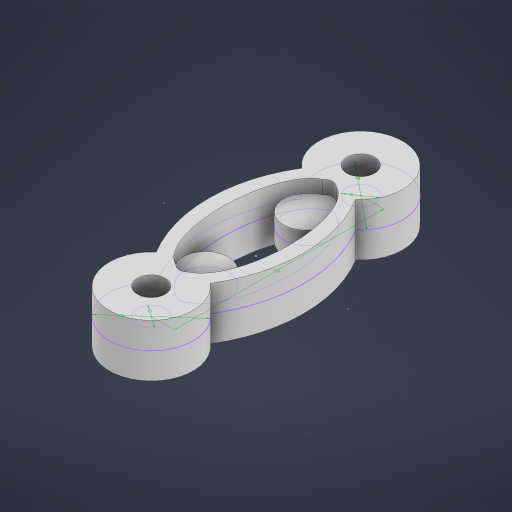
# Autodesk Inventor part: Part_A
Saved by Autodesk Inventor 2024.3 (Build 283343000, 343)
## iProperties
Created: 2025-07-11
Part Number: Part_A
Material: Generic
Document SubType Name: Modeling
Designer: LeoFB
Density: 1 g/cm^3
Appearance: Default
Author: LeoFB
Autodesk Inventor part; units mm, degrees
ref_plane "YZ Plane" through (0, 0, 0) normal (1, 0, 0) x (0, 1, 0)
ref_plane "XZ Plane" through (0, 0, 0) normal (0, 1, 0) x (-1, 0, 0)
ref_plane "XY Plane" through (0, 0, 0) normal (0, 0, 1) x (1, 0, 0)
sketch "Sketch1" plane through (0, 0, 0) normal (0, 1, 0) x (-1, 0, 0)
  circle A0 centre (0, 60) radius 8
  circle A1 centre (0, -60) radius 8
  arc A2 (15.4616, 41.6441) -> (-15.4616, 41.6441) centre (0, 60) ccw
  arc A3 (-15.4616, -41.6441) -> (15.4616, -41.6441) centre (0, -60) ccw
  arc A4 (15.4616, -41.6441) -> (15.4616, 41.6441) centre (-52.6044, 0) ccw
  arc A5 (-15.4616, 41.6441) -> (-15.4616, -41.6441) centre (52.6044, 0) ccw
  arc A6 (3.8493, 42.1449) -> (-3.8493, 42.1449) centre (0, 38.9538) ccw
  arc A7 (-3.8493, -42.1449) -> (3.8493, -42.1449) centre (0, -38.9538) ccw
  ellipse E0 centre (0, 0) end of major axis (0, 43.0192) minor radius 19.1905 (3.8493, -42.1449) -> (3.8493, 42.1449) ccw
  ellipse E1 centre (0, 0) end of major axis (0, 43.0192) minor radius 19.1905 (-3.8493, 42.1449) -> (-3.8493, -42.1449) ccw
  arc A8 (12.3481, -32.9308) -> (-12.3481, -32.9308) centre (0, -28.8656) ccw
  arc A9 (-12.3481, 32.9308) -> (12.3481, 32.9308) centre (0, 28.8656) ccw
  point P0 (-12.3481, 32.9308)
  point P1 (12.3481, 32.9308)
  dimension "d0" = 16
  dimension "d1" = 16
  dimension "d2" = 120
  dimension "d4" = 48
  dimension "d5" = 48
  constraints: 16 point on circle, 10 centre point, 3 coincident, 10 other
  measures "d0" diameter of A0
  measures "d1" diameter of A1
  measures "d2" distance of A1.centre A0.centre
  measures "d4" diameter of A2
  measures "d5" diameter of A3
extrude "Extrusion2" add sketch "Sketch1" along normal mid plane 30
extrude "Extrusion3" add sketch "Sketch1" along normal mid plane 15 contours E0 A9 E1 A6 | E0 A7 E1 A8
body "Solid2"
